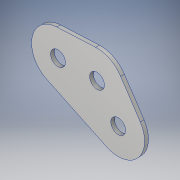
# Autodesk Inventor part: Gearbob Plate
Saved by Autodesk Inventor 2019.4 (Build 234330000, 330)
## iProperties
Created: 2019-11-02
Part Number: Gearbob Plate
Material: Aluminum 6061
Document SubType Name: Modeling
Designer: admin
Density: 2.7 g/cm^3
Appearance: Aluminum - Flat
Author: admin
Autodesk Inventor part; units mm, degrees
ref_plane "YZ Plane" through (0, 0, 0) normal (1, 0, 0) x (0, 1, 0)
ref_plane "XZ Plane" through (0, 0, 0) normal (0, 1, 0) x (-1, 0, 0)
ref_plane "XY Plane" through (0, 0, 0) normal (0, 0, 1) x (1, 0, 0)
sketch "Sketch1" plane through (0, 0, 0) normal (0, 0, 1) x (1, 0, 0)
  circle A0 centre (0, 0) radius 9.8
  circle A1 centre (51.75, 0) radius 9.8
  circle A2 centre (79.8368, -37.996) radius 9.8
  line L0 (0, 0) -> (51.75, 0) construction
  line L1 (79.8368, -37.996) -> (51.75, 0) construction
  arc A3 (109.0433, -18.7093) -> (64.796, -69.5994) centre (79.8368, -37.996) ccw construction
  arc A4 (49.9384, 37.4562) -> (83.0427, 20.6643) centre (51.75, 0) ccw construction
  arc A5 (-15.0407, -31.6034) -> (-1.6908, 34.9591) centre (0, 0) ccw construction
  line L2 (-1.6908, 34.9591) -> (49.9384, 37.4562)
  line L3 (83.0427, 20.6643) -> (109.0433, -18.7093)
  line L4 (64.796, -69.5994) -> (-15.0407, -31.6034)
  arc A6 (-1.6908, 34.9591) -> (-15.0407, -31.6034) centre (0, 0) ccw
  arc A7 (83.0427, 20.6643) -> (49.9384, 37.4562) centre (51.75, 0) ccw
  arc A8 (64.796, -69.5994) -> (109.0433, -18.7093) centre (79.8368, -37.996) ccw
  dimension "d0" = 19.6
  dimension "d1" = 19.6
  dimension "d2" = 19.6
  dimension "d3" = 51.75
  dimension "d4" = 47.25
  dimension "d5" = 37.996
  dimension "d6" = 70
  dimension "d7" = 75
  dimension "d8" = 70
  constraints: 12 point on circle, 10 end point, 9 centre point, 6 tangent, 4 coincident, 1 horizontal
  measures "d0" diameter of A0
  measures "d1" diameter of A1
  measures "d2" diameter of A2
  measures "d3" distance of L0.start L0.end
  measures "d4" distance of L1.start L0.end
  measures "d5" vertical distance of L1.start L0.end
  measures "d6" diameter of A3
  measures "d7" diameter of A4
  measures "d8" diameter of A5
extrude "Extrusion1" add sketch "Sketch1" along normal blind 5
body "Solid1"
